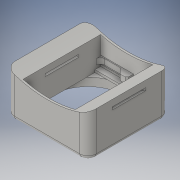
# Autodesk Inventor part: Christine Final
Saved by Autodesk Inventor 2016 (Build 200138000, 138)
## iProperties
Created: 2016-05-27
Part Number: Christine Final
Material: Generic
Document SubType Name: Modeling
Designer: xdlea
Density: 1 g/cm^3
Appearance: Default
LowerArch: 0.323 in
Height: 0.426 in
Width: 1.615 in
Length: 2.392 in
Author: xdlea
Autodesk Inventor part; units mm, degrees
note: some values were not read from the file. Chosen so that the rebuilt part matches the saved one: edges of "Fillet2".
ref_plane "YZ Plane" through (0, 0, 0) normal (1, 0, 0) x (0, 1, 0)
ref_plane "XZ Plane" through (0, 0, 0) normal (0, 1, 0) x (-1, 0, 0)
sketch "Sketch1" plane through (0, 0, 0) normal (0, 1, 0) x (-1, 0, 0)
  line L0 (-20.5105, 30.3784) -> (20.5105, 30.3784)
  line L1 (20.5105, 30.3784) -> (20.5105, 25.9334)
  line L2 (20.5105, -30.3784) -> (-20.5105, -30.3784)
  line L3 (-20.5105, -30.3784) -> (-20.5105, -25.9334)
  line L4 (-20.5105, 30.3784) -> (20.5105, -30.3784) construction
  line L5 (20.5105, 30.3784) -> (-20.5105, -30.3784) construction
  circle A0 centre (0, 0) radius 27.94 construction
  line L6 (-31.9659, 31.9659) -> (31.9659, 31.9659)
  line L7 (31.9659, 31.9659) -> (31.9659, -31.9659)
  line L8 (31.9659, -31.9659) -> (-31.9659, -31.9659)
  line L9 (-31.9659, -31.9659) -> (-31.9659, 31.9659)
  line L10 (-31.9659, 31.9659) -> (31.9659, -31.9659) construction
  line L11 (31.9659, 31.9659) -> (-31.9659, -31.9659) construction
  line L12 (20.5105, 25.9334) -> (-20.5105, 25.9334)
  line L13 (-20.5105, -25.9334) -> (20.5105, -25.9334)
  line L14 (20.5105, 25.9334) -> (20.5105, -25.9334)
  line L15 (-20.5105, 25.9334) -> (-20.5105, 30.3784)
  line L16 (-20.5105, -25.9334) -> (-20.5105, 25.9334)
  line L17 (20.5105, -25.9334) -> (20.5105, -30.3784)
  dimension "d0" = 41.021
  dimension "d1" = 60.7568
  dimension "d2" = 55.88
  dimension "d3" = 1.5875
  dimension "d4" = 4.445
  dimension "d5" = 4.445
  dimension "d43" = 63.9318
  constraints: 36 end point, 12 parallel, 11 perpendicular, 4 midpoint, 2 horizontal, 1 centre point, 1 coincident, 1 point on line
  measures "d0" distance of L2.start L2.end
  measures "d1" distance of L0.end L2.start
  measures "d2" diameter of A0
  measures "d3" distance between parallel lines of L6 L0
  measures "d4" distance between parallel lines of L2 L13
  measures "d5" distance between parallel lines of L12 L0
  measures "d43" distance of L6.end L7.end
extrude "Extrusion1" add sketch "Sketch1" against normal blind 1.905 contours L0 L1 L12 L15 | L13 L17 L2 L3 | L6 L7 L8 L9
extrude "Extrusion2" add sketch "Sketch1" along normal blind 10.795
sketch "Sketch2" plane through (0, -1.905, 0) normal (0, -1, 0) x (1, 0, 0)
  line L0 (31.9659, -31.9659) -> (31.9659, 31.9659) projected
  line L1 (31.9659, 31.9659) -> (-31.9659, 31.9659) projected
  line L2 (-31.9659, -31.9659) -> (31.9659, -31.9659) projected
  line L3 (-31.9659, 31.9659) -> (-31.9659, -31.9659) projected
  circle A0 centre (0, 0) radius 28.321
  dimension "d10" = 56.642
  constraints: 1 centre point, 1 coincident
  measures "d10" diameter of A0
extrude "Extrusion3" add sketch "Sketch2" along normal blind 6.35
fillet "Fillet1" radius 3.175 4 edges at (0, -8.255, -31.9659) (-31.9659, -8.255, 0) (0, -8.255, 31.9659) (31.9659, -8.255, 0)
sketch "Sketch3" plane through (-20.5105, 0, -30.3784) normal (0, 0, 1) x (1, 0, 0)
  line L0 (52.4764, 0) -> (-11.4554, 0) projected
  line L1 (18.6055, 6.9215) -> (24.9555, 6.9215)
  line L2 (24.9555, 6.9215) -> (24.9555, 2.4765)
  line L3 (24.9555, 2.4765) -> (18.6055, 2.4765)
  line L4 (18.6055, 2.4765) -> (18.6055, 6.9215)
  line L5 (18.6055, 6.9215) -> (24.9555, 2.4765) construction
  line L6 (24.9555, 6.9215) -> (18.6055, 2.4765) construction
  line L7 (0, 0) -> (0, 10.795) projected
  line L8 (0, 7.7153) -> (25.7493, 7.7153)
  line L9 (25.7493, 7.7153) -> (25.7493, 1.6828)
  line L10 (25.7493, 1.6828) -> (0, 1.6827)
  line L11 (0, 7.7153) -> (0, 6.9215)
  line L12 (18.6055, 6.9215) -> (0, 6.9215)
  line L13 (18.6055, 2.4765) -> (0, 2.4765)
  line L14 (0, 1.6827) -> (0, 2.4765)
  point P0 (20.5105, 0)
  point P1 (21.7805, 4.699)
  dimension "d14" = 21.7805
  dimension "d15" = 4.699
  dimension "d16" = 4.445
  dimension "d17" = 6.35
  dimension "d18" = 0.7937
  dimension "d19" = 0.7937
  dimension "d20" = 0.7937
  constraints: 26 end point, 6 perpendicular, 4 point on line, 2 horizontal, 2 midpoint, 2 parallel
  measures "d14" distance from line of L7 point (21.781, 4.699)
  measures "d15" distance from line of L0 point (21.781, 4.699)
  measures "d16" distance of L3.end L1.start
  measures "d17" distance of L2.end L3.end
  measures "d18" distance between parallel lines of L8 L1
  measures "d19" distance between parallel lines of L3 L10
  measures "d20" distance between parallel lines of L2 L9
extrude "Extrusion4" add sketch "Sketch3" along normal blind 4.445 contours L1 L2 L3 L4
extrude "Extrusion5" cut sketch "Sketch3" against normal up to next contours L12 L7 L8 L9 L10 L13 L3 L2 L1
chamfer "Chamfer1" distance 3.175 angle 45 1 edges at (-1.905, 4.699, -30.3784)
chamfer "Chamfer2" distance 1.27 angle 45 2 edges at (4.445, 4.699, -25.9334) (-1.905, 4.699, -25.9334)
sketch "Sketch4" plane through (31.9659, 10.795, -31.9659) normal (0, 0, -1) x (-1, 0, 0)
  line L0 (27.5209, -3.8735) -> (27.5209, -8.3185) projected
  line L1 (27.5209, -8.3185) -> (52.4764, -8.3185) projected
  line L2 (27.5209, -8.3185) -> (33.8709, -8.3185)
  line L3 (33.8709, -8.3185) -> (33.8709, -3.8735)
  line L4 (33.8709, -3.8735) -> (27.5209, -3.8735)
  point P0 (31.9659, -10.795)
  dimension "d31" = 6.35
  constraints: 6 end point, 1 perpendicular, 1 point on line, 1 vertical
  measures "d31" distance of L3.end L0.start
extrude "Extrusion6" add sketch "Sketch4" along normal blind 3.175
chamfer "Chamfer3" distance 1.27 angle 45 4 edges at (4.445, 4.699, -35.1409) (-1.905, 4.699, -35.1409) (1.27, 2.4765, -35.1409) (1.27, 6.9215, -35.1409)
fillet "Fillet2" radius 3.175 1 edges at (-20.5105, 4.699, -30.3784)
ref_plane "Work Plane1" through (-31.9659, 10.795, 0) normal (0, 0, 1) x (1, 0, 0)
sketch "Sketch5" plane through (-31.9659, 10.795, 0) normal (0, 0, 1) x (1, 0, 0)
  line L0 (52.4764, -10.795) -> (52.4764, 0) projected
  line L1 (52.4764, 0) -> (52.4764, 4.0194)
  arc A0 (52.4764, 4.0194) -> (63.9318, 7.62) centre (31.9659, 89.2966) ccw
  line L2 (0, 0) -> (63.9318, 0) projected
  line L3 (63.9318, 7.62) -> (63.9318, 0)
  line L4 (52.4764, 0) -> (63.9318, 0)
  line L5 (11.4554, -10.795) -> (11.4554, 0) projected
  line L6 (11.4554, 0) -> (11.4554, 4.0194)
  line L7 (0, 0) -> (0, 7.62)
  line L8 (11.4554, 0) -> (0, 0)
  arc A1 (0, 7.62) -> (11.4554, 4.0194) centre (31.9659, 89.2966) ccw
  arc A2 (0, 7.62) -> (63.9318, 7.62) centre (31.9659, 89.2966) ccw construction
  line L9 (52.4764, 4.0194) -> (52.4764, 5.9878)
  line L10 (11.4554, 4.0194) -> (11.4554, 5.9878)
  line L11 (0, 7.62) -> (0, 9.6774)
  line L12 (63.9318, 7.62) -> (63.9318, 9.6774)
  arc A3 (52.4764, 5.9878) -> (63.9318, 9.6774) centre (31.9659, 89.2966) ccw
  arc A4 (0, 9.6774) -> (11.4554, 5.9878) centre (31.9659, 89.2966) ccw
  line L13 (63.9318, 9.6774) -> (63.9318, 14.7574)
  line L14 (52.4764, 5.9878) -> (52.4764, 10.8286)
  line L15 (11.4554, 5.9878) -> (11.4554, 10.8286)
  line L16 (0, 9.6774) -> (0, 14.7574)
  arc A5 (52.4764, 10.8286) -> (63.9318, 14.7574) centre (31.9659, 89.2966) ccw
  arc A6 (0, 14.7574) -> (11.4554, 10.8286) centre (31.9659, 89.2966) ccw
  arc A7 (11.4554, 10.8286) -> (52.4764, 10.8286) centre (31.9659, 89.2966) ccw
  line L17 (11.4554, 0) -> (52.4764, 0)
  point P0 (31.9659, -10.795)
  point P1 (31.9659, 1.5875)
  point P2 (31.9659, 8.1923)
  dimension "d39" = 1.5875
  dimension "d40" = 7.62
  dimension "d41" = 2.0574
  dimension "d42" = 5.08
  dimension "d51" = 10.8286
  dimension "d52" = 41.021
  dimension "d53" = 8.1923
  constraints: 30 end point, 18 point on circle, 11 vertical, 8 centre point, 6 coincident, 6 parallel, 2 collinear, 1 concentric, 1 horizontal, 1 perpendicular
  measures "d39" distance from line of L2 point (31.966, 1.587)
  measures "d40" distance of L3.start L2.end
  measures "d41" distance of L3.start L12.end
  measures "d42" distance of L11.end L16.end
  measures "d51" distance from line of L2 L14.end
  measures "d52" distance of L5.end L0.end
  measures "d53" distance from line of L17 point (31.966, 8.192)
extrude "Extrusion7" add sketch "Sketch5" along normal mid plane 63.9318
extrude "Extrusion8" cut sketch "Sketch5" along normal mid plane 26.162 contours L9 A3 L12 A0 | A1 L11 A4 L10
extrude "Extrusion9" cut sketch "Sketch5" along normal mid plane 60.7568 contours L2 L6 L10 L15 A7 L14 L9 L1
fillet "Fillet3" radius 6.35 8 edges at (31.036, -7.3251, 31.036) (31.9659, 10.2362, 31.9659) (-31.036, -7.3251, 31.036) (-31.9659, 10.2362, 31.9659) (31.036, -7.3251, -31.036) (31.9659, 10.2362, -31.9659) (-31.036, -7.3251, -31.036) (-31.9659, 10.2362, -31.9659)
equation "\"d44\" = d43"
equation "\"d48\" = d1"
equation "\"LowerArch\" = d53"
equation "\"Height\" = d51"
equation "\"Width\" = d52"
equation "\"Length\" = d1"
body "Solid1"
